Autodesk Inventor part; units mm, degrees
(part 2 of 2)
  spline S29 degree 3 poles (15.4595, 40.7542) (15.3028, 40.5932) (15.0676, 40.3516) (14.7701, 40.0148) (14.5529, 39.757) (14.343, 39.4932) (14.1408, 39.2235) (13.9471, 38.9476) (13.763, 38.6652) (13.59, 38.3759) (13.4289, 38.0796) (13.3109, 37.8247) (13.221, 37.6188) (13.1407, 37.4703) (13.0453, 37.3311) (12.9327, 37.205) (12.8234, 37.1162) (12.7287, 37.0553) (12.6521, 37.02) (12.5744, 36.987) (12.4923, 36.9675) (12.4095, 36.9509) (12.3251, 36.9486) (12.2407, 36.9494) (12.1297, 36.9689) (11.993, 37.0006) (11.8552, 37.0273) (11.7459, 37.0546) (11.6684, 37.0882) (11.5922, 37.1246) (11.5234, 37.1735) (11.4563, 37.2247) (11.3987, 37.2864) (11.3431, 37.3498) (11.2814, 37.444) (11.2176, 37.5696) (11.166, 37.7306) (11.1355, 37.8966) (11.1225, 38.0648) (11.1242, 38.2895) (11.12, 38.5704) (11.0934, 38.9066) (11.0531, 39.2412) (10.9997, 39.5741) (10.935, 39.905) (10.86, 40.2336) (10.7755, 40.5599) (10.682, 40.8838) (10.5471, 41.3125) (10.4306, 41.6288) (10.3529, 41.8397) knots -1.0784 -1.0784 -1.0784 -1.0784 -1.010995 -0.977291 -0.943586 -0.909882 -0.876178 -0.842474 -0.80877 -0.775067 -0.741365 -0.707665 -0.690816 -0.67397 -0.657123 -0.640284 -0.623449 -0.615023 -0.606598 -0.598176 -0.589749 -0.581327 -0.572901 -0.564477 -0.556053 -0.5392 -0.522347 -0.513923 -0.505499 -0.497074 -0.488651 -0.480225 -0.471802 -0.463377 -0.454951 -0.438116 -0.421277 -0.40443 -0.387584 -0.370735 -0.337035 -0.303333 -0.26963 -0.235926 -0.202222 -0.168518 -0.134814 -0.101109 -0.067405 0 0 0 0 construction
  arc A24 (10.3529, 41.8397) -> (8.8856, 41.9939) centre (6.2752, 10.1006) ccw construction
  spline S30 degree 3 poles (8.8856, 41.9939) (8.7657, 41.8038) (8.5859, 41.5186) (8.3649, 41.1273) (8.2061, 40.83) (8.0556, 40.5283) (7.9139, 40.2225) (7.7818, 39.9123) (7.6604, 39.5978) (7.5514, 39.2789) (7.4554, 38.9556) (7.393, 38.6817) (7.3479, 38.4615) (7.3002, 38.2997) (7.2358, 38.1436) (7.1519, 37.9969) (7.0634, 37.8873) (6.9835, 37.808) (6.9159, 37.7576) (6.8467, 37.7092) (6.7704, 37.673) (6.6929, 37.6395) (6.6108, 37.6197) (6.5281, 37.603) (6.4155, 37.599) (6.2752, 37.6016) (6.1348, 37.599) (6.0223, 37.603) (5.9395, 37.6197) (5.8574, 37.6395) (5.7799, 37.673) (5.7037, 37.7092) (5.6344, 37.7576) (5.5669, 37.808) (5.487, 37.8873) (5.3985, 37.9969) (5.3146, 38.1436) (5.2502, 38.2997) (5.2025, 38.4615) (5.1574, 38.6817) (5.0949, 38.9556) (4.999, 39.2789) (4.89, 39.5978) (4.7685, 39.9123) (4.6365, 40.2225) (4.4948, 40.5283) (4.3443, 40.83) (4.1855, 41.1273) (3.9644, 41.5186) (3.7847, 41.8038) (3.6648, 41.9939) knots -1.0784 -1.0784 -1.0784 -1.0784 -1.010995 -0.977291 -0.943586 -0.909882 -0.876178 -0.842474 -0.80877 -0.775067 -0.741365 -0.707665 -0.690816 -0.67397 -0.657123 -0.640284 -0.623449 -0.615023 -0.606598 -0.598176 -0.589749 -0.581327 -0.572901 -0.564477 -0.556053 -0.5392 -0.522347 -0.513923 -0.505499 -0.497074 -0.488651 -0.480225 -0.471802 -0.463377 -0.454951 -0.438116 -0.421277 -0.40443 -0.387584 -0.370735 -0.337035 -0.303333 -0.26963 -0.235926 -0.202222 -0.168518 -0.134814 -0.101109 -0.067405 0 0 0 0 construction
  arc A25 (3.6648, 41.9939) -> (2.1975, 41.8397) centre (6.2752, 10.1006) ccw construction
  spline S31 degree 3 poles (2.1975, 41.8397) (2.1198, 41.6288) (2.0033, 41.3125) (1.8684, 40.8838) (1.7749, 40.5599) (1.6904, 40.2336) (1.6154, 39.905) (1.5507, 39.5741) (1.4973, 39.2412) (1.457, 38.9066) (1.4303, 38.5704) (1.4262, 38.2895) (1.4279, 38.0648) (1.4149, 37.8966) (1.3843, 37.7306) (1.3327, 37.5696) (1.269, 37.444) (1.2073, 37.3498) (1.1517, 37.2864) (1.0941, 37.2247) (1.027, 37.1735) (0.9581, 37.1246) (0.8819, 37.0882) (0.8045, 37.0546) (0.6952, 37.0273) (0.5574, 37.0006) (0.4207, 36.9689) (0.3097, 36.9494) (0.2253, 36.9486) (0.1409, 36.9509) (0.0581, 36.9675) (-0.024, 36.987) (-0.1018, 37.02) (-0.1784, 37.0553) (-0.273, 37.1162) (-0.3823, 37.205) (-0.4949, 37.3311) (-0.5904, 37.4703) (-0.6706, 37.6188) (-0.7605, 37.8247) (-0.8786, 38.0796) (-1.0396, 38.3759) (-1.2126, 38.6652) (-1.3967, 38.9476) (-1.5904, 39.2235) (-1.7926, 39.4932) (-2.0025, 39.757) (-2.2197, 40.0148) (-2.5173, 40.3516) (-2.7524, 40.5932) (-2.9091, 40.7542) knots -1.0784 -1.0784 -1.0784 -1.0784 -1.010995 -0.977291 -0.943586 -0.909882 -0.876178 -0.842474 -0.80877 -0.775067 -0.741365 -0.707665 -0.690816 -0.67397 -0.657123 -0.640284 -0.623449 -0.615023 -0.606598 -0.598176 -0.589749 -0.581327 -0.572901 -0.564477 -0.556053 -0.5392 -0.522347 -0.513923 -0.505499 -0.497074 -0.488651 -0.480225 -0.471802 -0.463377 -0.454951 -0.438116 -0.421277 -0.40443 -0.387584 -0.370735 -0.337035 -0.303333 -0.26963 -0.235926 -0.202222 -0.168518 -0.134814 -0.101109 -0.067405 0 0 0 0 construction
  arc A26 (-2.9091, 40.7542) -> (-4.3123, 40.2983) centre (6.2752, 10.1006) ccw construction
  spline S32 degree 3 poles (-4.3123, 40.2983) (-4.3445, 40.0759) (-4.3927, 39.7423) (-4.4355, 39.2948) (-4.4596, 38.9586) (-4.4744, 38.6219) (-4.4795, 38.2848) (-4.474, 37.9478) (-4.457, 37.6111) (-4.4268, 37.2753) (-4.383, 36.941) (-4.3286, 36.6653) (-4.2803, 36.4459) (-4.258, 36.2786) (-4.2534, 36.1099) (-4.2704, 35.9417) (-4.3066, 35.8056) (-4.3474, 35.7007) (-4.3886, 35.6271) (-4.4321, 35.5547) (-4.4871, 35.4907) (-4.5443, 35.4286) (-4.6112, 35.3771) (-4.68, 35.3282) (-4.7812, 35.2787) (-4.9105, 35.224) (-5.0377, 35.1646) (-5.1421, 35.1224) (-5.2245, 35.104) (-5.3075, 35.0887) (-5.392, 35.0878) (-5.4764, 35.0898) (-5.5593, 35.1059) (-5.6415, 35.1245) (-5.7468, 35.1644) (-5.8722, 35.2286) (-6.0085, 35.3285) (-6.1308, 35.4448) (-6.2402, 35.5733) (-6.371, 35.7561) (-6.5394, 35.9809) (-6.7586, 36.2372) (-6.9879, 36.4842) (-7.2267, 36.7222) (-7.4735, 36.9518) (-7.7274, 37.1736) (-7.9876, 37.3879) (-8.2536, 37.5949) (-8.6147, 37.8625) (-8.8949, 38.0499) (-9.0817, 38.1748) knots -1.0784 -1.0784 -1.0784 -1.0784 -1.010995 -0.977291 -0.943586 -0.909882 -0.876178 -0.842474 -0.80877 -0.775067 -0.741365 -0.707665 -0.690816 -0.67397 -0.657123 -0.640284 -0.623449 -0.615023 -0.606598 -0.598176 -0.589749 -0.581327 -0.572901 -0.564477 -0.556053 -0.5392 -0.522347 -0.513923 -0.505499 -0.497074 -0.488651 -0.480225 -0.471802 -0.463377 -0.454951 -0.438116 -0.421277 -0.40443 -0.387584 -0.370735 -0.337035 -0.303333 -0.26963 -0.235926 -0.202222 -0.168518 -0.134814 -0.101109 -0.067405 0 0 0 0 construction
  arc A27 (-9.0817, 38.1748) -> (-10.3594, 37.4372) centre (6.2752, 10.1006) ccw construction
  spline S33 degree 3 poles (-10.3594, 37.4372) (-10.3446, 37.2129) (-10.3225, 36.8766) (-10.2712, 36.43) (-10.225, 36.0961) (-10.1694, 35.7636) (-10.1043, 35.4329) (-10.0288, 35.1044) (-9.9422, 34.7786) (-9.8429, 34.4564) (-9.7305, 34.1385) (-9.6201, 33.8802) (-9.5272, 33.6756) (-9.4706, 33.5166) (-9.431, 33.3525) (-9.4126, 33.1845) (-9.4197, 33.0438) (-9.4378, 32.9327) (-9.4628, 32.8522) (-9.4904, 32.7723) (-9.5308, 32.6982) (-9.5739, 32.6256) (-9.6286, 32.5613) (-9.6857, 32.4992) (-9.7745, 32.4298) (-9.8895, 32.3494) (-10.0015, 32.2648) (-10.095, 32.2018) (-10.1717, 32.1667) (-10.2498, 32.1345) (-10.3322, 32.116) (-10.4151, 32.1005) (-10.4996, 32.0989) (-10.5839, 32.1) (-10.6951, 32.1172) (-10.8311, 32.1539) (-10.9853, 32.2232) (-11.1291, 32.3116) (-11.2628, 32.4146) (-11.4287, 32.5661) (-11.6402, 32.751) (-11.9078, 32.9562) (-12.1836, 33.1501) (-12.4666, 33.3332) (-12.7558, 33.5065) (-13.0502, 33.6706) (-13.3492, 33.8262) (-13.6525, 33.9734) (-14.0613, 34.1601) (-14.3744, 34.2851) (-14.5831, 34.3685) knots -1.0784 -1.0784 -1.0784 -1.0784 -1.010995 -0.977291 -0.943586 -0.909882 -0.876178 -0.842474 -0.80877 -0.775067 -0.741365 -0.707665 -0.690816 -0.67397 -0.657123 -0.640284 -0.623449 -0.615023 -0.606598 -0.598176 -0.589749 -0.581327 -0.572901 -0.564477 -0.556053 -0.5392 -0.522347 -0.513923 -0.505499 -0.497074 -0.488651 -0.480225 -0.471802 -0.463377 -0.454951 -0.438116 -0.421277 -0.40443 -0.387584 -0.370735 -0.337035 -0.303333 -0.26963 -0.235926 -0.202222 -0.168518 -0.134814 -0.101109 -0.067405 0 0 0 0 construction
  arc A28 (-14.5831, 34.3685) -> (-15.6795, 33.3813) centre (6.2752, 10.1006) ccw construction
  spline S34 degree 3 poles (-15.6795, 33.3813) (-15.6184, 33.165) (-15.5268, 32.8406) (-15.3839, 32.4145) (-15.2692, 32.0975) (-15.1457, 31.7838) (-15.0133, 31.4738) (-14.8711, 31.1682) (-14.7187, 30.8675) (-14.5546, 30.573) (-14.3785, 30.2854) (-14.2168, 30.0557) (-14.0834, 29.8749) (-13.9949, 29.7312) (-13.9221, 29.5789) (-13.8692, 29.4184) (-13.8469, 29.2793) (-13.8415, 29.1669) (-13.8492, 29.0829) (-13.8596, 28.9991) (-13.8838, 28.9182) (-13.9107, 28.8382) (-13.9509, 28.7639) (-13.9939, 28.6912) (-14.0662, 28.6049) (-14.1621, 28.5023) (-14.2541, 28.3963) (-14.3323, 28.3153) (-14.4001, 28.265) (-14.4698, 28.2173) (-14.5465, 28.1821) (-14.6244, 28.1496) (-14.7067, 28.1305) (-14.7894, 28.1141) (-14.9018, 28.1077) (-15.0425, 28.1153) (-15.2077, 28.1512) (-15.3667, 28.2077) (-15.5189, 28.2806) (-15.7127, 28.3944) (-15.958, 28.5312) (-16.2625, 28.6763) (-16.5725, 28.8087) (-16.8874, 28.9289) (-17.2063, 29.0383) (-17.5284, 29.1376) (-17.8532, 29.2276) (-18.1805, 29.3085) (-18.6192, 29.4061) (-18.9514, 29.4633) (-19.1729, 29.5015) knots -1.0784 -1.0784 -1.0784 -1.0784 -1.010995 -0.977291 -0.943586 -0.909882 -0.876178 -0.842474 -0.80877 -0.775067 -0.741365 -0.707665 -0.690816 -0.67397 -0.657123 -0.640284 -0.623449 -0.615023 -0.606598 -0.598176 -0.589749 -0.581327 -0.572901 -0.564477 -0.556053 -0.5392 -0.522347 -0.513923 -0.505499 -0.497074 -0.488651 -0.480225 -0.471802 -0.463377 -0.454951 -0.438116 -0.421277 -0.40443 -0.387584 -0.370735 -0.337035 -0.303333 -0.26963 -0.235926 -0.202222 -0.168518 -0.134814 -0.101109 -0.067405 0 0 0 0 construction
  arc A29 (-19.1729, 29.5015) -> (-20.0401, 28.3079) centre (6.2752, 10.1006) ccw construction
  spline S35 degree 3 poles (-20.0401, 28.3079) (-19.9354, 28.109) (-19.7783, 27.8108) (-19.5499, 27.4237) (-19.3718, 27.1375) (-19.1858, 26.8563) (-18.9918, 26.5807) (-18.7892, 26.3112) (-18.5776, 26.0488) (-18.3559, 25.7949) (-18.1239, 25.5502) (-17.9179, 25.3591) (-17.7498, 25.21) (-17.6334, 25.0878) (-17.5305, 24.954) (-17.4454, 24.808) (-17.3947, 24.6765) (-17.366, 24.5677) (-17.3561, 24.484) (-17.3488, 24.3998) (-17.3556, 24.3157) (-17.3654, 24.2318) (-17.3893, 24.1508) (-17.4162, 24.0708) (-17.469, 23.9713) (-17.5414, 23.8511) (-17.6093, 23.7282) (-17.6691, 23.6328) (-17.7249, 23.5695) (-17.7831, 23.5083) (-17.8509, 23.4579) (-17.9203, 23.4099) (-17.9969, 23.3742) (-18.0744, 23.3409) (-18.1829, 23.3113) (-18.3221, 23.2895) (-18.4911, 23.2902) (-18.6585, 23.3124) (-18.8225, 23.3521) (-19.0357, 23.4231) (-19.3041, 23.5059) (-19.6321, 23.5845) (-19.9628, 23.6495) (-20.2959, 23.7016) (-20.6305, 23.7424) (-20.9662, 23.7726) (-21.3027, 23.793) (-21.6396, 23.8042) (-22.0891, 23.8084) (-22.4259, 23.7953) (-22.6505, 23.7866) knots -1.0784 -1.0784 -1.0784 -1.0784 -1.010995 -0.977291 -0.943586 -0.909882 -0.876178 -0.842474 -0.80877 -0.775067 -0.741365 -0.707665 -0.690816 -0.67397 -0.657123 -0.640284 -0.623449 -0.615023 -0.606598 -0.598176 -0.589749 -0.581327 -0.572901 -0.564477 -0.556053 -0.5392 -0.522347 -0.513923 -0.505499 -0.497074 -0.488651 -0.480225 -0.471802 -0.463377 -0.454951 -0.438116 -0.421277 -0.40443 -0.387584 -0.370735 -0.337035 -0.303333 -0.26963 -0.235926 -0.202222 -0.168518 -0.134814 -0.101109 -0.067405 0 0 0 0 construction
  arc A30 (-22.6505, 23.7866) -> (-23.2505, 22.4388) centre (6.2752, 10.1006) ccw construction
  spline S36 degree 3 poles (-23.2505, 22.4388) (-23.1068, 22.266) (-22.8911, 22.0069) (-22.5872, 21.6758) (-22.3535, 21.4329) (-22.1132, 21.1965) (-21.8661, 20.9672) (-21.6119, 20.7458) (-21.3503, 20.5332) (-21.0807, 20.3309) (-20.8029, 20.1397) (-20.5616, 19.9957) (-20.3662, 19.8848) (-20.227, 19.7894) (-20.0985, 19.68) (-19.9849, 19.5548) (-19.908, 19.4368) (-19.8573, 19.3363) (-19.8302, 19.2564) (-19.8056, 19.1757) (-19.7947, 19.0919) (-19.7868, 19.0079) (-19.7934, 18.9237) (-19.803, 18.8398) (-19.834, 18.7315) (-19.8798, 18.5988) (-19.9208, 18.4646) (-19.9594, 18.3587) (-20.0008, 18.2852) (-20.045, 18.2133) (-20.1008, 18.1499) (-20.1588, 18.0885) (-20.2262, 18.0377) (-20.2951, 17.989) (-20.3951, 17.9375) (-20.5267, 17.8872) (-20.6922, 17.8527) (-20.8605, 17.8397) (-21.0292, 17.8444) (-21.2525, 17.8695) (-21.5323, 17.8948) (-21.8694, 17.9034) (-22.2064, 17.8983) (-22.5431, 17.88) (-22.8788, 17.8503) (-23.2135, 17.81) (-23.5469, 17.7601) (-23.8787, 17.7009) (-24.3192, 17.6116) (-24.646, 17.5288) (-24.8638, 17.4735) knots -1.0784 -1.0784 -1.0784 -1.0784 -1.010995 -0.977291 -0.943586 -0.909882 -0.876178 -0.842474 -0.80877 -0.775067 -0.741365 -0.707665 -0.690816 -0.67397 -0.657123 -0.640284 -0.623449 -0.615023 -0.606598 -0.598176 -0.589749 -0.581327 -0.572901 -0.564477 -0.556053 -0.5392 -0.522347 -0.513923 -0.505499 -0.497074 -0.488651 -0.480225 -0.471802 -0.463377 -0.454951 -0.438116 -0.421277 -0.40443 -0.387584 -0.370735 -0.337035 -0.303333 -0.26963 -0.235926 -0.202222 -0.168518 -0.134814 -0.101109 -0.067405 0 0 0 0 construction
  arc A31 (-24.8638, 17.4735) -> (-25.1706, 16.0304) centre (6.2752, 10.1006) ccw construction
  spline S37 degree 3 poles (-25.1706, 16.0304) (-24.9941, 15.8913) (-24.7292, 15.6827) (-24.3631, 15.422) (-24.084, 15.233) (-23.7998, 15.0518) (-23.5104, 14.8789) (-23.2158, 14.7151) (-22.9157, 14.5615) (-22.6099, 14.4197) (-22.2984, 14.2905) (-22.0325, 14.1998) (-21.8183, 14.1319) (-21.6623, 14.0676) (-21.5139, 13.9872) (-21.3767, 13.8884) (-21.2769, 13.789) (-21.2065, 13.7012) (-21.1633, 13.6287) (-21.1224, 13.5548) (-21.0945, 13.4752) (-21.0693, 13.3946) (-21.0581, 13.3109) (-21.0502, 13.2269) (-21.058, 13.1145) (-21.0752, 12.9752) (-21.0873, 12.8353) (-21.103, 12.7238) (-21.1283, 12.6433) (-21.1566, 12.5637) (-21.198, 12.4901) (-21.2419, 12.418) (-21.2973, 12.3543) (-21.3545, 12.2923) (-21.4417, 12.2211) (-21.56, 12.1446) (-21.7147, 12.0765) (-21.8766, 12.0287) (-22.0426, 11.9983) (-22.2662, 11.9764) (-22.5451, 11.9429) (-22.8767, 11.8813) (-23.2053, 11.8062) (-23.5308, 11.7183) (-23.853, 11.6194) (-24.172, 11.5105) (-24.4877, 11.3923) (-24.8, 11.2655) (-25.2123, 11.0865) (-25.5147, 10.9376) (-25.7163, 10.8382) knots -1.0784 -1.0784 -1.0784 -1.0784 -1.010995 -0.977291 -0.943586 -0.909882 -0.876178 -0.842474 -0.80877 -0.775067 -0.741365 -0.707665 -0.690816 -0.67397 -0.657123 -0.640284 -0.623449 -0.615023 -0.606598 -0.598176 -0.589749 -0.581327 -0.572901 -0.564477 -0.556053 -0.5392 -0.522347 -0.513923 -0.505499 -0.497074 -0.488651 -0.480225 -0.471802 -0.463377 -0.454951 -0.438116 -0.421277 -0.40443 -0.387584 -0.370735 -0.337035 -0.303333 -0.26963 -0.235926 -0.202222 -0.168518 -0.134814 -0.101109 -0.067405 0 0 0 0 construction
  arc A32 (-25.7163, 10.8382) -> (-25.7163, 9.3629) centre (6.2752, 10.1006) ccw construction
  spline S38 degree 3 poles (-25.7163, 9.3629) (-25.5147, 9.2636) (-25.2123, 9.1146) (-24.8, 8.9357) (-24.4877, 8.8088) (-24.172, 8.6906) (-23.853, 8.5817) (-23.5308, 8.4828) (-23.2053, 8.3949) (-22.8767, 8.3198) (-22.5451, 8.2582) (-22.2662, 8.2247) (-22.0426, 8.2028) (-21.8766, 8.1724) (-21.7147, 8.1246) (-21.56, 8.0565) (-21.4417, 7.98) (-21.3545, 7.9088) (-21.2973, 7.8469) (-21.2419, 7.7831) (-21.198, 7.711) (-21.1566, 7.6374) (-21.1283, 7.5578) (-21.103, 7.4773) (-21.0873, 7.3658) (-21.0752, 7.2259) (-21.058, 7.0866) (-21.0502, 6.9742) (-21.0581, 6.8902) (-21.0693, 6.8065) (-21.0945, 6.7259) (-21.1224, 6.6463) (-21.1633, 6.5724) (-21.2065, 6.4999) (-21.2769, 6.4121) (-21.3767, 6.3127) (-21.5139, 6.2139) (-21.6623, 6.1335) (-21.8183, 6.0692) (-22.0325, 6.0013) (-22.2984, 5.9106) (-22.6099, 5.7814) (-22.9157, 5.6396) (-23.2158, 5.486) (-23.5104, 5.3222) (-23.7998, 5.1493) (-24.084, 4.9681) (-24.3631, 4.7791) (-24.7292, 4.5184) (-24.9941, 4.3098) (-25.1706, 4.1707) knots -1.0784 -1.0784 -1.0784 -1.0784 -1.010995 -0.977291 -0.943586 -0.909882 -0.876178 -0.842474 -0.80877 -0.775067 -0.741365 -0.707665 -0.690816 -0.67397 -0.657123 -0.640284 -0.623449 -0.615023 -0.606598 -0.598176 -0.589749 -0.581327 -0.572901 -0.564477 -0.556053 -0.5392 -0.522347 -0.513923 -0.505499 -0.497074 -0.488651 -0.480225 -0.471802 -0.463377 -0.454951 -0.438116 -0.421277 -0.40443 -0.387584 -0.370735 -0.337035 -0.303333 -0.26963 -0.235926 -0.202222 -0.168518 -0.134814 -0.101109 -0.067405 0 0 0 0 construction
  arc A33 (-25.1706, 4.1707) -> (-24.8638, 2.7276) centre (6.2752, 10.1006) ccw construction
  spline S39 degree 3 poles (-24.8638, 2.7276) (-24.646, 2.6724) (-24.3192, 2.5895) (-23.8787, 2.5002) (-23.5469, 2.4411) (-23.2135, 2.3911) (-22.8788, 2.3509) (-22.5431, 2.3211) (-22.2064, 2.3028) (-21.8694, 2.2977) (-21.5323, 2.3063) (-21.2525, 2.3316) (-21.0292, 2.3567) (-20.8605, 2.3614) (-20.6922, 2.3484) (-20.5267, 2.3139) (-20.3951, 2.2636) (-20.2951, 2.2121) (-20.2262, 2.1635) (-20.1588, 2.1126) (-20.1008, 2.0512) (-20.045, 1.9878) (-20.0008, 1.9159) (-19.9594, 1.8424) (-19.9208, 1.7366) (-19.8798, 1.6023) (-19.834, 1.4696) (-19.803, 1.3613) (-19.7934, 1.2774) (-19.7868, 1.1933) (-19.7947, 1.1092) (-19.8056, 1.0255) (-19.8302, 0.9447) (-19.8573, 0.8648) (-19.908, 0.7643) (-19.9849, 0.6463) (-20.0985, 0.5212) (-20.227, 0.4117) (-20.3662, 0.3163) (-20.5616, 0.2054) (-20.8029, 0.0614) (-21.0807, -0.1298) (-21.3503, -0.332) (-21.6119, -0.5447) (-21.8661, -0.7661) (-22.1132, -0.9954) (-22.3535, -1.2318) (-22.5872, -1.4747) (-22.8911, -1.8058) (-23.1068, -2.0649) (-23.2505, -2.2376) knots -1.0784 -1.0784 -1.0784 -1.0784 -1.010995 -0.977291 -0.943586 -0.909882 -0.876178 -0.842474 -0.80877 -0.775067 -0.741365 -0.707665 -0.690816 -0.67397 -0.657123 -0.640284 -0.623449 -0.615023 -0.606598 -0.598176 -0.589749 -0.581327 -0.572901 -0.564477 -0.556053 -0.5392 -0.522347 -0.513923 -0.505499 -0.497074 -0.488651 -0.480225 -0.471802 -0.463377 -0.454951 -0.438116 -0.421277 -0.40443 -0.387584 -0.370735 -0.337035 -0.303333 -0.26963 -0.235926 -0.202222 -0.168518 -0.134814 -0.101109 -0.067405 0 0 0 0 construction
  arc A34 (-23.2505, -2.2376) -> (-22.6505, -3.5855) centre (6.2752, 10.1006) ccw construction
  spline S40 degree 3 poles (-22.6505, -3.5855) (-22.4259, -3.5942) (-22.0891, -3.6073) (-21.6396, -3.6031) (-21.3027, -3.5919) (-20.9662, -3.5715) (-20.6305, -3.5413) (-20.2959, -3.5005) (-19.9628, -3.4484) (-19.6321, -3.3834) (-19.3041, -3.3048) (-19.0357, -3.222) (-18.8225, -3.151) (-18.6585, -3.1113) (-18.4911, -3.0891) (-18.3221, -3.0884) (-18.1829, -3.1102) (-18.0744, -3.1398) (-17.9969, -3.173) (-17.9203, -3.2088) (-17.8509, -3.2568) (-17.7831, -3.3072) (-17.7249, -3.3683) (-17.6691, -3.4316) (-17.6093, -3.5271) (-17.5414, -3.65) (-17.469, -3.7702) (-17.4162, -3.8697) (-17.3893, -3.9497) (-17.3654, -4.0307) (-17.3556, -4.1146) (-17.3488, -4.1987) (-17.3561, -4.2829) (-17.366, -4.3666) (-17.3947, -4.4754) (-17.4454, -4.6069) (-17.5305, -4.7529) (-17.6334, -4.8867) (-17.7498, -5.0089) (-17.9179, -5.158) (-18.1239, -5.3491) (-18.3559, -5.5938) (-18.5776, -5.8477) (-18.7892, -6.1101) (-18.9918, -6.3795) (-19.1858, -6.6552) (-19.3718, -6.9364) (-19.5499, -7.2226) (-19.7783, -7.6097) (-19.9354, -7.9079) (-20.0401, -8.1068) knots -1.0784 -1.0784 -1.0784 -1.0784 -1.010995 -0.977291 -0.943586 -0.909882 -0.876178 -0.842474 -0.80877 -0.775067 -0.741365 -0.707665 -0.690816 -0.67397 -0.657123 -0.640284 -0.623449 -0.615023 -0.606598 -0.598176 -0.589749 -0.581327 -0.572901 -0.564477 -0.556053 -0.5392 -0.522347 -0.513923 -0.505499 -0.497074 -0.488651 -0.480225 -0.471802 -0.463377 -0.454951 -0.438116 -0.421277 -0.40443 -0.387584 -0.370735 -0.337035 -0.303333 -0.26963 -0.235926 -0.202222 -0.168518 -0.134814 -0.101109 -0.067405 0 0 0 0 construction
  arc A35 (-20.0401, -8.1068) -> (-19.1729, -9.3004) centre (6.2752, 10.1006) ccw construction
  spline S41 degree 3 poles (-19.1729, -9.3004) (-18.9514, -9.2622) (-18.6192, -9.205) (-18.1805, -9.1074) (-17.8532, -9.0265) (-17.5284, -8.9365) (-17.2063, -8.8372) (-16.8874, -8.7278) (-16.5725, -8.6075) (-16.2625, -8.4751) (-15.958, -8.3301) (-15.7127, -8.1933) (-15.5189, -8.0795) (-15.3667, -8.0066) (-15.2077, -7.95) (-15.0425, -7.9142) (-14.9018, -7.9066) (-14.7894, -7.913) (-14.7067, -7.9294) (-14.6244, -7.9485) (-14.5465, -7.981) (-14.4698, -8.0162) (-14.4001, -8.0639) (-14.3323, -8.1142) (-14.2541, -8.1952) (-14.1621, -8.3012) (-14.0662, -8.4038) (-13.9939, -8.4901) (-13.9509, -8.5628) (-13.9107, -8.637) (-13.8838, -8.7171) (-13.8596, -8.7979) (-13.8492, -8.8818) (-13.8415, -8.9657) (-13.8469, -9.0782) (-13.8692, -9.2173) (-13.9221, -9.3778) (-13.9949, -9.5301) (-14.0834, -9.6738) (-14.2168, -9.8546) (-14.3785, -10.0843) (-14.5546, -10.3719) (-14.7187, -10.6664) (-14.8711, -10.9671) (-15.0133, -11.2727) (-15.1457, -11.5827) (-15.2692, -11.8964) (-15.3839, -12.2133) (-15.5268, -12.6395) (-15.6184, -12.9639) (-15.6795, -13.1801) knots -1.0784 -1.0784 -1.0784 -1.0784 -1.010995 -0.977291 -0.943586 -0.909882 -0.876178 -0.842474 -0.80877 -0.775067 -0.741365 -0.707665 -0.690816 -0.67397 -0.657123 -0.640284 -0.623449 -0.615023 -0.606598 -0.598176 -0.589749 -0.581327 -0.572901 -0.564477 -0.556053 -0.5392 -0.522347 -0.513923 -0.505499 -0.497074 -0.488651 -0.480225 -0.471802 -0.463377 -0.454951 -0.438116 -0.421277 -0.40443 -0.387584 -0.370735 -0.337035 -0.303333 -0.26963 -0.235926 -0.202222 -0.168518 -0.134814 -0.101109 -0.067405 0 0 0 0 construction
  arc A36 (-15.6795, -13.1801) -> (-14.5831, -14.1674) centre (6.2752, 10.1006) ccw construction
  spline S42 degree 3 poles (-14.5831, -14.1674) (-14.3744, -14.084) (-14.0613, -13.959) (-13.6525, -13.7723) (-13.3492, -13.6251) (-13.0502, -13.4695) (-12.7558, -13.3054) (-12.4666, -13.1321) (-12.1836, -12.949) (-11.9078, -12.7551) (-11.6402, -12.5499) (-11.4287, -12.365) (-11.2628, -12.2134) (-11.1291, -12.1105) (-10.9853, -12.0221) (-10.8311, -11.9528) (-10.6951, -11.9161) (-10.5839, -11.8989) (-10.4996, -11.8978) (-10.4151, -11.8993) (-10.3322, -11.9149) (-10.2498, -11.9334) (-10.1717, -11.9656) (-10.095, -12.0007) (-10.0015, -12.0637) (-9.8895, -12.1482) (-9.7745, -12.2287) (-9.6857, -12.2981) (-9.6286, -12.3602) (-9.5739, -12.4245) (-9.5308, -12.4971) (-9.4904, -12.5712) (-9.4628, -12.6511) (-9.4378, -12.7316) (-9.4197, -12.8427) (-9.4126, -12.9834) (-9.431, -13.1514) (-9.4706, -13.3155) (-9.5272, -13.4745) (-9.6201, -13.6791) (-9.7305, -13.9374) (-9.8429, -14.2553) (-9.9422, -14.5775) (-10.0288, -14.9033) (-10.1043, -15.2318) (-10.1694, -15.5625) (-10.225, -15.895) (-10.2712, -16.2289) (-10.3225, -16.6754) (-10.3446, -17.0118) (-10.3594, -17.236) knots -1.0784 -1.0784 -1.0784 -1.0784 -1.010995 -0.977291 -0.943586 -0.909882 -0.876178 -0.842474 -0.80877 -0.775067 -0.741365 -0.707665 -0.690816 -0.67397 -0.657123 -0.640284 -0.623449 -0.615023 -0.606598 -0.598176 -0.589749 -0.581327 -0.572901 -0.564477 -0.556053 -0.5392 -0.522347 -0.513923 -0.505499 -0.497074 -0.488651 -0.480225 -0.471802 -0.463377 -0.454951 -0.438116 -0.421277 -0.40443 -0.387584 -0.370735 -0.337035 -0.303333 -0.26963 -0.235926 -0.202222 -0.168518 -0.134814 -0.101109 -0.067405 0 0 0 0 construction
  arc A37 (-10.3594, -17.236) -> (-9.0817, -17.9737) centre (6.2752, 10.1006) ccw construction
  spline S43 degree 3 poles (-9.0817, -17.9737) (-8.8949, -17.8488) (-8.6147, -17.6614) (-8.2536, -17.3938) (-7.9876, -17.1868) (-7.7274, -16.9724) (-7.4735, -16.7507) (-7.2267, -16.521) (-6.9879, -16.2831) (-6.7586, -16.0361) (-6.5394, -15.7798) (-6.371, -15.5549) (-6.2402, -15.3722) (-6.1308, -15.2437) (-6.0085, -15.1273) (-5.8722, -15.0274) (-5.7468, -14.9633) (-5.6415, -14.9234) (-5.5593, -14.9048) (-5.4764, -14.8887) (-5.392, -14.8867) (-5.3075, -14.8876) (-5.2245, -14.9029) (-5.1421, -14.9213) (-5.0377, -14.9634) (-4.9105, -15.0229) (-4.7812, -15.0776) (-4.68, -15.1271) (-4.6112, -15.176) (-4.5443, -15.2274) (-4.4871, -15.2896) (-4.4321, -15.3536) (-4.3886, -15.426) (-4.3474, -15.4996) (-4.3066, -15.6045) (-4.2704, -15.7406) (-4.2534, -15.9088) (-4.258, -16.0775) (-4.2803, -16.2448) (-4.3286, -16.4642) (-4.383, -16.7399) (-4.4268, -17.0742) (-4.457, -17.41) (-4.474, -17.7467) (-4.4795, -18.0837) (-4.4744, -18.4208) (-4.4596, -18.7575) (-4.4355, -19.0937) (-4.3927, -19.5412) (-4.3445, -19.8748) (-4.3123, -20.0972) knots -1.0784 -1.0784 -1.0784 -1.0784 -1.010995 -0.977291 -0.943586 -0.909882 -0.876178 -0.842474 -0.80877 -0.775067 -0.741365 -0.707665 -0.690816 -0.67397 -0.657123 -0.640284 -0.623449 -0.615023 -0.606598 -0.598176 -0.589749 -0.581327 -0.572901 -0.564477 -0.556053 -0.5392 -0.522347 -0.513923 -0.505499 -0.497074 -0.488651 -0.480225 -0.471802 -0.463377 -0.454951 -0.438116 -0.421277 -0.40443 -0.387584 -0.370735 -0.337035 -0.303333 -0.26963 -0.235926 -0.202222 -0.168518 -0.134814 -0.101109 -0.067405 0 0 0 0 construction
  arc A38 (-4.3123, -20.0972) -> (-2.9091, -20.5531) centre (6.2752, 10.1006) ccw construction
  spline S44 degree 3 poles (-2.9091, -20.5531) (-2.7524, -20.3921) (-2.5173, -20.1505) (-2.2197, -19.8137) (-2.0025, -19.5559) (-1.7926, -19.2921) (-1.5904, -19.0224) (-1.3967, -18.7465) (-1.2126, -18.4641) (-1.0396, -18.1748) (-0.8786, -17.8785) (-0.7605, -17.6236) (-0.6706, -17.4176) (-0.5904, -17.2692) (-0.4949, -17.13) (-0.3823, -17.0039) (-0.273, -16.9151) (-0.1784, -16.8542) (-0.1018, -16.8189) (-0.024, -16.7859) (0.0581, -16.7664) (0.1409, -16.7498) (0.2253, -16.7475) (0.3097, -16.7483) (0.4207, -16.7678) (0.5574, -16.7995) (0.6952, -16.8262) (0.8045, -16.8535) (0.8819, -16.887) (0.9581, -16.9235) (1.027, -16.9723) (1.0941, -17.0236) (1.1517, -17.0853) (1.2073, -17.1487) (1.269, -17.2428) (1.3327, -17.3685) (1.3843, -17.5294) (1.4149, -17.6954) (1.4279, -17.8637) (1.4262, -18.0884) (1.4303, -18.3693) (1.457, -18.7055) (1.4973, -19.0401) (1.5507, -19.373) (1.6154, -19.7038) (1.6904, -20.0325) (1.7749, -20.3588) (1.8684, -20.6826) (2.0033, -21.1114) (2.1198, -21.4277) (2.1975, -21.6386) knots -1.0784 -1.0784 -1.0784 -1.0784 -1.010995 -0.977291 -0.943586 -0.909882 -0.876178 -0.842474 -0.80877 -0.775067 -0.741365 -0.707665 -0.690816 -0.67397 -0.657123 -0.640284 -0.623449 -0.615023 -0.606598 -0.598176 -0.589749 -0.581327 -0.572901 -0.564477 -0.556053 -0.5392 -0.522347 -0.513923 -0.505499 -0.497074 -0.488651 -0.480225 -0.471802 -0.463377 -0.454951 -0.438116 -0.421277 -0.40443 -0.387584 -0.370735 -0.337035 -0.303333 -0.26963 -0.235926 -0.202222 -0.168518 -0.134814 -0.101109 -0.067405 0 0 0 0 construction
  arc A39 (2.1975, -21.6386) -> (3.6648, -21.7928) centre (6.2752, 10.1006) ccw construction
  spline S45 degree 3 poles (3.6648, -21.7928) (3.7847, -21.6027) (3.9644, -21.3175) (4.1855, -20.9262) (4.3443, -20.6289) (4.4948, -20.3272) (4.6365, -20.0214) (4.7685, -19.7112) (4.89, -19.3967) (4.999, -19.0777) (5.0949, -18.7545) (5.1574, -18.4806) (5.2025, -18.2604) (5.2502, -18.0985) (5.3146, -17.9425) (5.3985, -17.7958) (5.487, -17.6862) (5.5669, -17.6069) (5.6344, -17.5565) (5.7037, -17.5081) (5.7799, -17.4719) (5.8574, -17.4384) (5.9395, -17.4186) (6.0223, -17.4019) (6.1348, -17.3979) (6.2752, -17.4005) (6.4155, -17.3979) (6.5281, -17.4019) (6.6108, -17.4186) (6.6929, -17.4384) (6.7704, -17.4719) (6.8467, -17.5081) (6.9159, -17.5565) (6.9835, -17.6069) (7.0634, -17.6862) (7.1519, -17.7958) (7.2358, -17.9425) (7.3002, -18.0985) (7.3479, -18.2604) (7.393, -18.4806) (7.4554, -18.7545) (7.5514, -19.0777) (7.6604, -19.3967) (7.7818, -19.7112) (7.9139, -20.0214) (8.0556, -20.3272) (8.2061, -20.6289) (8.3649, -20.9262) (8.5859, -21.3175) (8.7657, -21.6027) (8.8856, -21.7928) knots -1.0784 -1.0784 -1.0784 -1.0784 -1.010995 -0.977291 -0.943586 -0.909882 -0.876178 -0.842474 -0.80877 -0.775067 -0.741365 -0.707665 -0.690816 -0.67397 -0.657123 -0.640284 -0.623449 -0.615023 -0.606598 -0.598176 -0.589749 -0.581327 -0.572901 -0.564477 -0.556053 -0.5392 -0.522347 -0.513923 -0.505499 -0.497074 -0.488651 -0.480225 -0.471802 -0.463377 -0.454951 -0.438116 -0.421277 -0.40443 -0.387584 -0.370735 -0.337035 -0.303333 -0.26963 -0.235926 -0.202222 -0.168518 -0.134814 -0.101109 -0.067405 0 0 0 0 construction
  arc A40 (8.8856, -21.7928) -> (10.3529, -21.6386) centre (6.2752, 10.1006) ccw construction
  circle A41 centre (6.2752, 10.1006) radius 4 construction
  arc A42 (-0.2248, -22.3994) -> (-3.4816, -28.2994) centre (6.3896, -29.8994) ccw construction
  arc A43 (-3.4816, -31.4994) -> (-3.4816, -28.2994) centre (-3.4785, -29.8994) ccw construction
  arc A44 (-3.4816, -31.4994) -> (-0.2248, -37.3994) centre (6.3896, -29.8994) ccw construction
  line L38 (-0.2248, -37.3994) -> (12.7752, -37.3994) construction
  arc A45 (12.7752, -37.3994) -> (16.0345, -31.4838) centre (6.1608, -29.8994) ccw construction
  arc A46 (16.0345, -28.3151) -> (16.0345, -31.4838) centre (16.2577, -29.8994) ccw construction
  arc A47 (16.0345, -28.3151) -> (12.7752, -22.3994) centre (6.1608, -29.8994) ccw construction
  line L39 (12.7752, -22.3994) -> (-0.2248, -22.3994) construction
  arc A48 (2.7045, -26.3994) -> (9.8459, -26.3994) centre (6.2752, -29.8994) ccw construction
  line L40 (2.7045, -26.3994) -> (9.8459, -26.3994) construction
  circle A49 centre (6.2752, 10.1006) radius 4.1
  arc A50 (-3.5992, -31.3946) -> (-0.2625, -37.4994) centre (6.3896, -29.8994) ccw
  arc A51 (-3.5992, -31.3946) -> (-3.5992, -28.4043) centre (-3.4785, -29.8994) ccw
  arc A52 (-0.2625, -22.2994) -> (-3.5992, -28.4043) centre (6.3896, -29.8994) ccw
  line L41 (-0.2625, -22.2994) -> (12.8129, -22.2994)
  arc A53 (16.1494, -28.4034) -> (12.8129, -22.2994) centre (6.1608, -29.8994) ccw
  arc A54 (16.1494, -28.4034) -> (16.1494, -31.3955) centre (16.2577, -29.8994) ccw
  arc A55 (12.8129, -37.4994) -> (16.1494, -31.3955) centre (6.1608, -29.8994) ccw
  line L42 (12.8129, -37.4994) -> (-0.2625, -37.4994)
  arc A56 (12.8129, -37.4994) -> (12.8129, -22.2994) centre (6.1608, -29.8994) ccw
  arc A57 (-0.2625, -22.2994) -> (-0.2625, -37.4994) centre (6.3896, -29.8994) ccw
  line L43 (29.0856, -48.6611) -> (19.0856, -48.6611)
  line L44 (19.0856, -48.6611) -> (19.0856, -38.6611)
  line L45 (19.0856, -38.6611) -> (29.0856, -38.6611)
  line L46 (29.0856, -38.6611) -> (29.0856, -48.6611)
  line L47 (0, -48.6611) -> (0, 58.6611) construction
  line L48 (-19.0856, -48.6611) -> (-19.0856, -38.6611)
  line L49 (-19.0856, -38.6611) -> (-29.0856, -38.6611)
  circle A58 centre (24.0856, -43.6611) radius 1.25
  circle A59 centre (-24.0854, -43.6611) radius 1.25
  circle A60 centre (24.0856, 53.6609) radius 1.25
  circle A61 centre (-24.0854, 53.6609) radius 1.25
  point P0 (-29.0854, 80.3446)
  dimension "d23" = 1
  dimension "d24" = 0.1
  dimension "d25" = 0.1
  dimension "d26" = 10
  dimension "d27" = 10
  dimension "d28" = 2.5
  dimension "d31" = 48.171
  dimension "d34" = 97.322
  constraints: 28 end point, 16 point on circle, 13 centre point, 4 parallel, 3 concentric, 3 horizontal, 3 perpendicular, 3 point on line, 3 symmetric about line, 2 midpoint, 1 vertical, 13 other
  measures "d23" distance between parallel lines of L25 L8
  measures "d24" radial gap between concentric circles of A41 A49
  measures "d25" radial gap between concentric circles of A44 A50
  measures "d26" distance of L44.end L45.end
  measures "d27" distance of L43.end L44.end
  measures "d28" diameter of A58
  measures "d31" distance of A58.centre A59.centre
  measures "d34" distance of A58.centre A60.centre
extrude "Extrusion3" add sketch "Sketch3" along normal blind 8 contours L4 L44 L45 L7 | L4 L5 L49 L48 | L8 L5 L6 L7 | A49
sketch "Sketch4" plane through (29.0854, -80.3446, 10) normal (0, 0, 1) x (1, 0, 0)
  arc A0 (-0.2248, -22.3994) -> (-3.4816, -28.2994) centre (6.3896, -29.8994) ccw construction
  arc A1 (-3.4816, -31.4994) -> (-3.4816, -28.2994) centre (-3.4785, -29.8994) ccw construction
  arc A2 (-3.4816, -31.4994) -> (-0.2248, -37.3994) centre (6.3896, -29.8994) ccw construction
  line L0 (-0.2248, -37.3994) -> (12.7752, -37.3994) construction
  arc A3 (12.7752, -37.3994) -> (16.0345, -31.4838) centre (6.1608, -29.8994) ccw construction
  arc A4 (16.0345, -28.3151) -> (16.0345, -31.4838) centre (16.2577, -29.8994) ccw construction
  arc A5 (16.0345, -28.3151) -> (12.7752, -22.3994) centre (6.1608, -29.8994) ccw construction
  line L1 (12.7752, -22.3994) -> (-0.2248, -22.3994) construction
  arc A6 (2.7045, -26.3994) -> (9.8459, -26.3994) centre (6.2752, -29.8994) ccw construction
  line L2 (2.7045, -26.3994) -> (9.8459, -26.3994) construction
  line L3 (29.0856, -48.6611) -> (29.0856, 58.6611) construction
  line L4 (29.0856, 58.6611) -> (-29.0856, 58.6611) construction
  line L5 (-29.0856, 58.6611) -> (-29.0856, -48.6611) construction
  line L6 (-29.0856, -48.6611) -> (29.0856, -48.6611) construction
  circle A7 centre (24.0856, -43.6611) radius 1.25 construction
  line L7 (29.0856, -48.6611) -> (29.0856, -38.6611) projected
  line L8 (-29.0856, 58.6611) -> (-29.0856, 48.6611) projected
  line L9 (29.0856, -48.6611) -> (-29.0856, -48.6611)
  line L10 (-29.0856, -48.6611) -> (-29.0856, 58.6611)
  line L11 (-29.0856, 58.6611) -> (29.0856, 58.6611)
  line L12 (29.0856, 58.6611) -> (29.0856, -48.6611)
  arc A8 (-3.5992, -31.3946) -> (-0.2625, -37.4994) centre (6.3896, -29.8994) ccw
  arc A9 (-3.5992, -31.3946) -> (-3.5992, -28.4043) centre (-3.4785, -29.8994) ccw
  arc A10 (-0.2625, -22.2994) -> (-3.5992, -28.4043) centre (6.3896, -29.8994) ccw
  line L13 (-0.2625, -22.2994) -> (12.8129, -22.2994)
  arc A11 (16.1494, -28.4034) -> (12.8129, -22.2994) centre (6.1608, -29.8994) ccw
  arc A12 (16.1494, -28.4034) -> (16.1494, -31.3955) centre (16.2577, -29.8994) ccw
  arc A13 (12.8129, -37.4994) -> (16.1494, -31.3955) centre (6.1608, -29.8994) ccw
  line L14 (12.8129, -37.4994) -> (-0.2625, -37.4994)
  arc A14 (12.8129, -37.4994) -> (12.8129, -22.2994) centre (6.1608, -29.8994) ccw
  arc A15 (-0.2625, -22.2994) -> (-0.2625, -37.4994) centre (6.3896, -29.8994) ccw
  circle A16 centre (24.0856, -43.6611) radius 1.25
  circle A17 centre (-24.0854, -43.6611) radius 1.25 projected
  circle A18 centre (24.0856, 53.6609) radius 1.25 projected
  circle A19 centre (-24.0854, 53.6609) radius 1.25 projected
  line L15 (24.0856, -17.2994) -> (-24.0856, -17.2994)
  line L16 (-24.0856, -17.2994) -> (-24.0856, 43.6611)
  line L17 (-24.0856, 43.6611) -> (24.0856, 43.6611)
  line L18 (24.0856, 43.6611) -> (24.0856, -17.2994)
  line L19 (-29.0856, 48.6611) -> (29.0856, 48.6611) projected
  circle A20 centre (6.2752, 10.1006) radius 4.1 projected
  line L20 (10.3752, 43.6611) -> (2.1752, 43.6611)
  line L21 (2.1752, 43.6611) -> (2.1752, -17.2994)
  line L22 (2.1752, -17.2994) -> (10.3752, -17.2994)
  line L23 (10.3752, -17.2994) -> (10.3752, 43.6611)
  line L24 (24.0856, 14.2006) -> (-24.0856, 14.2006)
  line L25 (-24.0856, 14.2006) -> (-24.0856, 6.0006)
  line L26 (-24.0856, 6.0006) -> (24.0856, 6.0006)
  line L27 (24.0856, 6.0006) -> (24.0856, 14.2006)
  point P0 (-29.0854, 80.3446)
  point P1 (2.1752, 14.2006)
  point P2 (10.3752, 14.2006)
  point P3 (10.3752, 6.0006)
  point P4 (24.0856, 6.0006)
  point P5 (10.3752, -17.2994)
  point P6 (13.2722, -22.7274)
  point P7 (12.887, -37.4339)
  point P8 (-3.5992, -31.3946)
  point P9 (-3.5992, -28.4043)
  point P10 (2.1752, 6.0006)
  dimension "d39" = 0.1
  dimension "d40" = 5
  dimension "d41" = 5
  dimension "d42" = 5
  dimension "d43" = 5
  constraints: 36 end point, 16 point on circle, 9 centre point, 8 parallel, 4 horizontal, 4 perpendicular, 4 point on line, 2 concentric, 1 coincident, 7 other
  measures "d39" radial gap between concentric circles of A2 A8
  measures "d40" distance between parallel lines of L17 L19
  measures "d41" distance between parallel lines of L3 L18
  measures "d42" distance between parallel lines of L5 L16
  measures "d43" distance from line of L13 L15.start
extrude "Extrusion4" add sketch "Sketch4" along normal blind 9.5 contours L9 L10 L19 L12 L7 | L19 L8 L11 L12 | L15 L21 L26 L23 | L26 L23 L24 L18 | L26 A20 L23 | L26 L16 L24 L21 | L21 A20 L26 | A20 | A20 L24 L23 | L24 L21 L17 L23 | L21 L24 A20
ref_plane "Work Plane3" through (61.7399, -126.5057, 16.9) normal (0, 0, -1) x (-1, 0, 0)
sketch "Sketch5" plane through (61.7399, -126.5057, 16.9) normal (0, 0, -1) x (-1, 0, 0)
  circle A0 centre (8.5689, 2.5) radius 1.25 projected
  circle A1 centre (8.5689, 2.5) radius 3
  line L0 (3.5689, -2.5) -> (3.5689, 104.8221) construction
  line L1 (3.5689, 104.8221) -> (61.7401, 104.8221) construction
  line L2 (61.7401, 104.8221) -> (61.7401, -2.5) construction
  line L3 (61.7401, -2.5) -> (3.5689, -2.5) construction
  line L4 (30.4793, 60.3616) -> (56.7401, 60.3616) construction
  line L5 (56.7401, 60.3616) -> (56.7401, 89.8221) construction
  line L6 (56.7401, 89.8221) -> (30.4793, 89.8221) construction
  line L7 (30.4793, 89.8221) -> (30.4793, 60.3616) construction
  line L8 (22.2793, 60.3616) -> (22.2793, 89.8221) construction
  line L9 (22.2793, 89.8221) -> (8.5689, 89.8221) construction
  line L10 (8.5689, 89.8221) -> (8.5689, 60.3616) construction
  line L11 (8.5689, 60.3616) -> (22.2793, 60.3616) construction
  line L12 (22.2793, 52.1616) -> (8.5689, 52.1616) construction
  line L13 (8.5689, 52.1616) -> (8.5689, 28.8616) construction
  line L14 (8.5689, 28.8616) -> (22.2793, 28.8616) construction
  line L15 (22.2793, 28.8616) -> (22.2793, 52.1616) construction
  line L16 (32.917, 23.8616) -> (19.8416, 23.8616) construction
  arc A2 (19.8416, 23.8616) -> (19.8417, 8.6616) centre (26.4937, 16.2616) ccw construction
  line L17 (19.8417, 8.6616) -> (32.917, 8.6616) construction
  arc A3 (32.917, 8.6616) -> (32.917, 23.8616) centre (26.265, 16.2616) ccw construction
  circle A4 centre (56.7399, 2.5) radius 1.25 construction
  circle A5 centre (8.5689, 2.5) radius 1.25 construction
  circle A6 centre (8.5689, 99.822) radius 1.25 construction
  circle A7 centre (56.7399, 99.822) radius 1.25 construction
  line L18 (30.4793, 52.1616) -> (30.4793, 28.8616) construction
  line L19 (30.4793, 28.8616) -> (56.7401, 28.8616) construction
  line L20 (56.7401, 28.8616) -> (56.7401, 52.1616) construction
  line L21 (56.7401, 52.1616) -> (30.4793, 52.1616) construction
  circle A8 centre (56.7399, 2.5) radius 3
  circle A9 centre (8.5689, 99.822) radius 3
  circle A10 centre (56.7399, 99.822) radius 3
  point P0 (61.7399, 126.5057)
  dimension "d46" = 6
  dimension "d49" = 48.171
  dimension "d52" = 97.322
  constraints: 4 centre point, 1 coincident, 1 horizontal, 1 vertical, 6 other
  measures "d46" diameter of A1
  measures "d49" distance of A1.centre A8.centre
  measures "d52" distance of A1.centre A9.centre
extrude "Extrusion5" cut sketch "Sketch5" against normal blind 26.25 contours A0 | A1 | A8 | A9 | A10
chamfer "Chamfer1" distance 1 angle 45 4 edges at (56.171, -124.0057, 19.5) (8, -124.0057, 19.5) (56.171, -26.6837, 19.5) (8, -26.6837, 19.5)
body "Solid2"
